Autodesk Fusion 360 part; units mm, degrees
(part 3 of 4)
sketch "Ultra96-V2" plane through (0, -0.5, 0) normal (0, -1, 0) x (1, 0, 0) in component "Card Plate"
  circle A0 centre (18.5, 38.5) radius 1.35
  circle A1 centre (18.5, -38.5) radius 1.35
  circle A2 centre (4, -38.5) radius 1.35
  circle A3 centre (4, 38.5) radius 1.35
  circle A4 centre (50, -38.5) radius 1.35
  circle A5 centre (81.5, 38.5) radius 1.35
  circle A6 centre (50, 38.5) radius 1.35
  circle A7 centre (81.5, -38.5) radius 1.35
  circle A8 centre (75, 46) radius 1.35
  circle A9 centre (17, -46) radius 1.35
  circle A10 centre (17, 46) radius 1.35
  circle A11 centre (75, -46) radius 1.35
  circle A12 centre (81.5, 24.5) radius 1.35
  circle A13 centre (81.5, -24.5) radius 1.35
  circle A14 centre (23.5, 24.5) radius 1.35
  circle A15 centre (23.5, -24.5) radius 1.35
  line L0 (100, 52) -> (15, 52)
  line L1 (15, 52) -> (15, 50)
  line L2 (15, 50) -> (0, 50)
  line L3 (0, 50) -> (0, -50)
  line L4 (0, -50) -> (15, -50)
  line L5 (15, -50) -> (15, -52)
  line L6 (15, -52) -> (100, -52)
  line L7 (100, -52) -> (100, 52)
  line L8 (0, 42.5) -> (54, 42.5) construction
  line L9 (54, 42.5) -> (54, -42.5) construction
  line L10 (54, -42.5) -> (0, -42.5) construction
  line L11 (0, -42.5) -> (0, 42.5) construction
  circle A16 centre (6, 17.5) radius 1.35
  circle A17 centre (48, 17.5) radius 1.35
  circle A18 centre (48, -24.5) radius 1.35
  circle A19 centre (6, -24.5) radius 1.35
  line L12 (6, 17.5) -> (48, 17.5) construction
  line L13 (48, 17.5) -> (48, -24.5) construction
  line L14 (48, -24.5) -> (6, -24.5) construction
  line L15 (6, -24.5) -> (6, 17.5) construction
  line L16 (31.5836, -52) -> (31.5836, -42.5) construction
  line L17 (34.961, 42.5) -> (34.961, 52) construction
  dimension "d222" = 54
  dimension "d223" = 85
  dimension "d224" = 2.7
  dimension "d225" = 2.7
  dimension "d226" = 2.7
  dimension "d227" = 2.7
  dimension "d228" = 42
  dimension "d229" = 42
  dimension "d231" = 18
  dimension "d232" = 6
  constraint horizontal L8
  constraint vertical L9
  constraint horizontal L10
  constraint vertical L11
  constraint collinear L3 L11
  constraint coincident A16.centre L12.start
  constraint coincident A17.centre L12.end
  constraint coincident A18.centre L13.end
  constraint vertical L13
  constraint coincident A19.centre L14.end
  constraint vertical L15
  constraint horizontal L12
  constraint horizontal L14
  constraint coincident L6 L16.start
  constraint coincident L10 L16.end
  constraint perpendicular L10 L16
  constraint coincident L8 L17.start
  constraint coincident L0 L17.end
  constraint perpendicular L0 L17
  constraint equal L16 L17
  measures "d222" distance of L8.start L8.end
  measures "d223" distance of L8.start L10.end
  measures "d224" diameter of A16
  measures "d225" diameter of A17
  measures "d226" diameter of A19
  measures "d227" diameter of A18
  measures "d228" distance of A16.centre A17.centre
  measures "d229" distance of A19.centre A16.centre
  measures "d231" distance of L10 A18.centre
  measures "d232" distance of L9 A18.centre
extrude "Extrude12" cut sketch "Ultra96-V2" against normal blind 8 contours A16 | A17 | A18 | A19 bodies 1 in component "Card Plate"
sketch "Jetson Nano" plane through (0, -0.5, 0) normal (0, -1, 0) x (1, 0, 0) in component "Card Plate"
  circle A0 centre (48, 17.5) radius 1.35
  circle A1 centre (48, -24.5) radius 1.35
  circle A2 centre (6, 17.5) radius 1.35
  circle A3 centre (6, -24.5) radius 1.35
  circle A4 centre (18.5, 38.5) radius 1.35
  circle A5 centre (18.5, -38.5) radius 1.35
  circle A6 centre (4, -38.5) radius 1.35
  circle A7 centre (4, 38.5) radius 1.35
  circle A8 centre (50, -38.5) radius 1.35
  circle A9 centre (81.5, 38.5) radius 1.35
  circle A10 centre (50, 38.5) radius 1.35
  circle A11 centre (81.5, -38.5) radius 1.35
  circle A12 centre (75, 46) radius 1.35
  circle A13 centre (17, -46) radius 1.35
  circle A14 centre (17, 46) radius 1.35
  circle A15 centre (75, -46) radius 1.35
  circle A16 centre (81.5, 24.5) radius 1.35
  circle A17 centre (81.5, -24.5) radius 1.35
  circle A18 centre (23.5, 24.5) radius 1.35
  circle A19 centre (23.5, -24.5) radius 1.35
  line L0 (100, 52) -> (15, 52)
  line L1 (15, 52) -> (15, 50)
  line L2 (15, 50) -> (0, 50)
  line L3 (0, 50) -> (0, -50)
  line L4 (0, -50) -> (15, -50)
  line L5 (15, -50) -> (15, -52)
  line L6 (15, -52) -> (100, -52)
  line L7 (100, -52) -> (100, 52)
  line L8 (0, 50) -> (79, 50) construction
  line L9 (79, 50) -> (79, -50) construction
  line L10 (79, -50) -> (0, -50) construction
  line L11 (0, -50) -> (0, 50) construction
  line L12 (29.4049, 50) -> (29.4049, 52) construction
  line L13 (32.781, -50) -> (32.781, -52) construction
  circle A20 centre (17, 46) radius 1.35
  circle A21 centre (75, 46) radius 1.35
  circle A22 centre (17, -40) radius 1.35
  circle A23 centre (75, -40) radius 1.35
  line L14 (17, 46) -> (75, 46) construction
  line L15 (75, 46) -> (75, -40) construction
  line L16 (75, -40) -> (17, -40) construction
  line L17 (17, -40) -> (17, 46) construction
  dimension "d235" = 79
  dimension "d236" = 100
  dimension "d237" = 2.7
  dimension "d238" = 2.7
  dimension "d239" = 2.7
  dimension "d240" = 2.7
  dimension "d241" = 17
  dimension "d242" = 4
  dimension "d243" = 86
  dimension "d244" = 58
  constraint horizontal L8
  constraint vertical L9
  constraint horizontal L10
  constraint vertical L11
  constraint coincident L8 L12.start
  constraint coincident L0 L12.end
  constraint perpendicular L0 L12
  constraint coincident L10 L13.start
  constraint coincident L6 L13.end
  constraint perpendicular L6 L13
  constraint equal L12 L13
  constraint collinear L3 L11
  constraint coincident A14.centre A20.centre
  constraint coincident A12.centre A21.centre
  constraint coincident A23.centre L15.end
  constraint coincident A22.centre L16.end
  constraint horizontal L14
  constraint vertical L15
  constraint vertical L17
  constraint horizontal L16
  measures "d235" distance of L2.end L8.end
  measures "d236" distance of L2.end L3.end
  measures "d237" diameter of A20
  measures "d238" diameter of A21
  measures "d239" diameter of A22
  measures "d240" diameter of A23
  measures "d241" distance of L11 A14.centre
  measures "d242" distance of L8 A14.centre
  measures "d243" distance of A14.centre A22.centre
  measures "d244" distance of A14.centre A12.centre
extrude "Extrude13" cut sketch "Jetson Nano" against normal blind 12 contours A5 A22 | A23 picked at (17.0516, -39.9573) bodies 1 in component "Card Plate"
sketch "SolidRun Hummingboard" plane through (0, -0.5, 0) normal (0, -1, 0) x (1, 0, 0) in component "Card Plate"
  line L0 (100, 52) -> (15, 52)
  line L1 (15, 52) -> (15, 50)
  line L2 (15, 50) -> (0, 50)
  line L3 (0, 50) -> (0, -50)
  line L4 (0, -50) -> (15, -50)
  line L5 (15, -50) -> (15, -52)
  line L6 (15, -52) -> (100, -52)
  line L7 (100, -52) -> (100, 52)
  circle A0 centre (23.5, -24.5) radius 1.35
  circle A1 centre (23.5, 24.5) radius 1.35
  circle A2 centre (81.5, -24.5) radius 1.35
  circle A3 centre (81.5, 24.5) radius 1.35
  circle A4 centre (75, -46) radius 1.35
  circle A5 centre (17, 46) radius 1.35
  circle A6 centre (17, -46) radius 1.35
  circle A7 centre (75, 46) radius 1.35
  circle A8 centre (81.5, -38.5) radius 1.35
  circle A9 centre (50, 38.5) radius 1.35
  circle A10 centre (81.5, 38.5) radius 1.35
  circle A11 centre (50, -38.5) radius 1.35
  circle A12 centre (4, 38.5) radius 1.35
  circle A13 centre (4, -38.5) radius 1.35
  arc A14 (17.1594, -38.6594) -> (18.3406, -39.8406) centre (17, -40) ccw
  arc A15 (18.3406, -39.8406) -> (17.1594, -38.6594) centre (18.5, -38.5) ccw
  circle A16 centre (18.5, 38.5) radius 1.35
  circle A17 centre (6, -24.5) radius 1.35
  circle A18 centre (6, 17.5) radius 1.35
  circle A19 centre (48, -24.5) radius 1.35
  circle A20 centre (48, 17.5) radius 1.35
  circle A21 centre (75, -40) radius 1.35
  line L8 (0, 50.959) -> (73, 50.959) construction
  line L9 (73, 50.959) -> (73, -49.041) construction
  line L10 (73, -49.041) -> (0, -49.041) construction
  line L11 (0, -49.041) -> (0, 50.959) construction
  circle A22 centre (2.838, 46.861) radius 1.35
  circle A23 centre (68.73, 48.639) radius 1.35
  circle A24 centre (68.73, -46.861) radius 1.35
  circle A25 centre (4.33, -46.861) radius 1.35
  line L12 (2.838, 46.861) -> (2.838, 50) construction
  line L13 (4.33, -46.861) -> (4.33, -50) construction
  dimension "d247" = 73
  dimension "d248" = 100
  dimension "d249" = 2.7
  dimension "d250" = 2.7
  dimension "d251" = 2.7
  dimension "d252" = 2.7
  dimension "d253" = 2.838
  dimension "d254" = 4.098
  dimension "d255" = 4.27
  dimension "d256" = 2.32
  dimension "d257" = 4.27
  dimension "d258" = 2.18
  dimension "d259" = 4.33
  dimension "d260" = 2.18
  constraint horizontal L8
  constraint vertical L9
  constraint horizontal L10
  constraint vertical L11
  constraint collinear L3 L11
  constraint coincident A22.centre L12.start
  constraint coincident L2 L12.end
  constraint perpendicular L2 L12
  constraint coincident A25.centre L13.start
  constraint coincident L4 L13.end
  constraint perpendicular L4 L13
  constraint equal L12 L13
  measures "d247" distance of L8.start L8.end
  measures "d248" distance of L8.start L10.end
  measures "d249" diameter of A22
  measures "d250" diameter of A23
  measures "d251" diameter of A24
  measures "d252" diameter of A25
  measures "d253" distance of L11 A22.centre
  measures "d254" distance of L8 A22.centre
  measures "d255" distance of L9 A23.centre
  measures "d256" distance of L8 A23.centre
  measures "d257" distance of L9 A24.centre
  measures "d258" distance of L10 A24.centre
  measures "d259" distance of L11 A25.centre
  measures "d260" distance of L10 A25.centre
extrude "Extrude14" cut sketch "SolidRun Hummingboard" against normal blind 55 contours A22 | A23 | A24 | A25 bodies 1 in component "Card Plate"
sketch "Cutout - Broad" plane through (0, -0.5, 0) normal (0, -1, 0) x (1, 0, 0) in component "Card Plate"
  circle A0 centre (68.73, 48.639) radius 1.35
  circle A1 centre (4.33, -46.861) radius 1.35
  circle A2 centre (2.838, 46.861) radius 1.35
  circle A3 centre (68.73, -46.861) radius 1.35
  line L0 (100, 52) -> (15, 52)
  line L1 (15, 52) -> (15, 50)
  line L2 (15, 50) -> (0, 50)
  line L3 (0, 50) -> (0, -50)
  line L4 (0, -50) -> (15, -50)
  line L5 (15, -50) -> (15, -52)
  line L6 (15, -52) -> (100, -52)
  line L7 (100, -52) -> (100, 52)
  circle A4 centre (23.5, -24.5) radius 1.35
  circle A5 centre (23.5, 24.5) radius 1.35
  circle A6 centre (81.5, -24.5) radius 1.35
  circle A7 centre (81.5, 24.5) radius 1.35
  circle A8 centre (75, -46) radius 1.35
  circle A9 centre (17, 46) radius 1.35
  circle A10 centre (17, -46) radius 1.35
  circle A11 centre (75, 46) radius 1.35
  circle A12 centre (81.5, -38.5) radius 1.35
  circle A13 centre (50, 38.5) radius 1.35
  circle A14 centre (81.5, 38.5) radius 1.35
  circle A15 centre (50, -38.5) radius 1.35
  circle A16 centre (4, 38.5) radius 1.35
  circle A17 centre (4, -38.5) radius 1.35
  arc A18 (17.1594, -38.6594) -> (18.3406, -39.8406) centre (17, -40) ccw
  arc A19 (18.3406, -39.8406) -> (17.1594, -38.6594) centre (18.5, -38.5) ccw
  circle A20 centre (18.5, 38.5) radius 1.35
  circle A21 centre (6, -24.5) radius 1.35
  circle A22 centre (6, 17.5) radius 1.35
  circle A23 centre (48, -24.5) radius 1.35
  circle A24 centre (48, 17.5) radius 1.35
  circle A25 centre (75, -40) radius 1.35
  line L8 (11, -33.5) -> (18.5, -33.5)
  line L9 (18.5, -33.5) -> (18.5, -19.5)
  line L10 (18.5, -19.5) -> (28.5, -19.5)
  line L11 (28.5, -19.5) -> (28.5, -47)
  line L12 (28.5, -47) -> (43, -47)
  line L13 (43, -47) -> (43, -19.5)
  line L14 (43, -19.5) -> (55, -19.5)
  line L15 (55, -19.5) -> (55, -47)
  line L16 (55, -47) -> (63.73, -47)
  line L17 (63.73, -47) -> (63.73, -44.9205)
  line L18 (63.73, -44.9205) -> (76.5, -30.9468)
  line L19 (76.5, -30.9468) -> (76.5, -18.1196)
  line L20 (76.5, -18.1196) -> (86.5, -18.1196)
  line L21 (86.5, -18.1196) -> (86.5, -47)
  line L22 (86.5, -47) -> (95, -47)
  line L23 (95, -47) -> (95, 47)
  line L24 (95, 47) -> (86.5, 47)
  line L25 (86.5, 47) -> (86.5, 19.5)
  line L26 (86.5, 19.5) -> (76.5, 19.5)
  line L27 (76.5, 19.5) -> (76.5, 39.9438)
  line L28 (76.5, 39.9438) -> (59.7352, 47)
  line L29 (59.7352, 47) -> (55, 47)
  line L30 (55, 47) -> (55, 12.5)
  line L31 (55, 12.5) -> (43, 12.5)
  line L32 (43, 12.5) -> (43, 47)
  line L33 (43, 47) -> (28.5, 47)
  line L34 (28.5, 47) -> (28.5, 19.5)
  line L35 (28.5, 19.5) -> (18.5, 19.5)
  line L36 (18.5, 19.5) -> (18.5, 33.5)
  line L37 (18.5, 33.5) -> (11, 33.5)
  line L38 (100, 52) -> (100, -52)
  line L39 (15, 52) -> (100, 52)
  line L40 (100, -52) -> (15, -52)
  line L41 (11, -33.5) -> (11, -19.5)
  line L42 (11, -19.5) -> (5, -19.5)
  line L43 (5, -19.5) -> (5, 12.5)
  line L44 (5, 12.5) -> (11, 12.5)
  line L45 (11, 12.5) -> (11, 33.5)
  dimension "d287" = 5
  dimension "d288" = 5
  dimension "d289" = 5
  dimension "d290" = 5
  dimension "d291" = 5
  dimension "d292" = 5
  dimension "d293" = 5
  dimension "d294" = 5
  dimension "d295" = 5
  dimension "d296" = 5
  dimension "d297" = 5
  dimension "d298" = 5
  dimension "d299" = 5
  dimension "d300" = 5
  dimension "d301" = 5
  dimension "d302" = 5
  dimension "d303" = 5
  dimension "d306" = 5
  dimension "d307" = 5
  dimension "d308" = 5
  dimension "d309" = 5
  dimension "d310" = 5
  dimension "d311" = 5
  dimension "d312" = 5
  dimension "d313" = 5
  dimension "d314" = 5
  dimension "d315" = 5
  dimension "d316" = 5
  dimension "d317" = 5
  dimension "d318" = 5
  dimension "d319" = 5
  dimension "d320" = 5
  dimension "d321" = 5
  dimension "d322" = 5
  dimension "d323" = 5
  dimension "d324" = 5
  constraint perpendicular L8 L9
  constraint perpendicular L9 L10
  constraint perpendicular L10 L11
  constraint perpendicular L11 L12
  constraint perpendicular L12 L13
  constraint perpendicular L13 L14
  constraint perpendicular L12 L15
  constraint perpendicular L15 L16
  constraint perpendicular L16 L17
  constraint perpendicular L16 L19
  constraint perpendicular L19 L20
  constraint perpendicular L20 L21
  constraint perpendicular L21 L22
  constraint perpendicular L22 L23
  constraint perpendicular L23 L24
  constraint perpendicular L24 L25
  constraint perpendicular L25 L26
  constraint perpendicular L26 L27
  constraint perpendicular L27 L29
  constraint perpendicular L29 L30
  constraint perpendicular L30 L31
  constraint perpendicular L29 L32
  constraint perpendicular L32 L33
  constraint perpendicular L33 L34
  constraint perpendicular L34 L35
  constraint perpendicular L33 L36
  constraint perpendicular L36 L37
  constraint perpendicular L8 L41
  constraint perpendicular L41 L42
  constraint perpendicular L42 L43
  constraint perpendicular L43 L44
  constraint perpendicular L37 L45
  measures "d287" distance of L23 L38
  measures "d288" distance of A6.centre L21
  measures "d289" distance of A7.centre L25
  measures "d290" distance of A7.centre L27
  measures "d291" distance of L29 L39
  measures "d292" distance of L33 L39
  measures "d293" distance of L16 L40
  measures "d294" distance of L12 L40
  measures "d295" distance of A3.centre L17
  measures "d296" distance of A6.centre L19
  measures "d297" distance of A25.centre L18
  measures "d298" distance of A3.centre L18
  measures "d299" distance of A13.centre L30
  measures "d300" distance of A24.centre L32
  measures "d301" distance of A5.centre L34
  measures "d302" distance of A5.centre L35
  measures "d303" distance of A20.centre L37
  measures "d306" distance of A4.centre L11
  measures "d307" distance of A15.centre L15
  measures "d308" distance of A23.centre L13
  measures "d309" distance of A4.centre L9
  measures "d310" distance of A4.centre L10
  measures "d311" distance of A19.centre L8
  measures "d312" distance of A0.centre L28
  measures "d313" distance of A11.centre L28
  measures "d314" distance of A7.centre L26
  measures "d315" distance of A24.centre L31
  measures "d316" distance of A23.centre L14
  measures "d317" distance of L22 L40
  measures "d318" distance of L24 L39
  measures "d319" distance of A22.centre L45
  measures "d320" distance of L3 L43
  measures "d321" distance of A21.centre L42
  measures "d322" distance of A21.centre L41
  measures "d323" distance of A5.centre L36
  measures "d324" distance of A22.centre L44
extrude "Extrude15" cut sketch "Cutout - Broad" against normal blind 20 contours L8 L9 L10 L11 L12 L13 L14 L15 L16 L17 L18 L19 L20 L21 L22 L23 L24 L25 L26 L27 L28 L29 L30 L31 L32 L33 L34 L35 L36 L37 L41 L42 L43 L44 L45 bodies 1 in component "Card Plate"
sketch "Cutout - Supports" plane through (0, -0.5, 0) normal (0, -1, 0) x (1, 0, 0) in component "Card Plate"
  line L0 (18.5, -19.5) -> (18.5, -33.5)
  line L1 (18.5, -33.5) -> (11, -33.5)
  line L2 (11, -33.5) -> (11, -19.5)
  line L3 (11, -19.5) -> (5, -19.5)
  line L4 (5, -19.5) -> (5, 12.5)
  line L5 (5, 12.5) -> (11, 12.5)
  line L6 (11, 12.5) -> (11, 33.5)
  line L7 (11, 33.5) -> (18.5, 33.5)
  line L8 (18.5, 33.5) -> (18.5, 19.5)
  line L9 (18.5, 19.5) -> (28.5, 19.5)
  line L10 (28.5, 19.5) -> (28.5, 47)
  line L11 (28.5, 47) -> (43, 47)
  line L12 (43, 47) -> (43, 12.5)
  line L13 (43, 12.5) -> (55, 12.5)
  line L14 (55, 12.5) -> (55, 47)
  line L15 (55, 47) -> (59.7352, 47)
  line L16 (59.7352, 47) -> (76.5, 39.9438)
  line L17 (76.5, 39.9438) -> (76.5, 19.5)
  line L18 (76.5, 19.5) -> (86.5, 19.5)
  line L19 (86.5, 19.5) -> (86.5, 47)
  line L20 (86.5, 47) -> (95, 47)
  line L21 (95, 47) -> (95, -47)
  line L22 (95, -47) -> (86.5, -47)
  line L23 (86.5, -47) -> (86.5, -18.1196)
  line L24 (86.5, -18.1196) -> (76.5, -18.1196)
  line L25 (76.5, -18.1196) -> (76.5, -30.9468)
  line L26 (76.5, -30.9468) -> (63.73, -44.9205)
  line L27 (63.73, -44.9205) -> (63.73, -47)
  line L28 (63.73, -47) -> (55, -47)
  line L29 (55, -47) -> (55, -19.5)
  line L30 (55, -19.5) -> (43, -19.5)
  line L31 (43, -19.5) -> (43, -47)
  line L32 (43, -47) -> (28.5, -47)
  line L33 (28.5, -47) -> (28.5, -19.5)
  line L34 (28.5, -19.5) -> (18.5, -19.5)
  circle A0 centre (68.73, 48.639) radius 1.35
  circle A1 centre (4.33, -46.861) radius 1.35
  circle A2 centre (2.838, 46.861) radius 1.35
  circle A3 centre (68.73, -46.861) radius 1.35
  line L35 (100, 52) -> (15, 52)
  line L36 (15, 52) -> (15, 50)
  line L37 (15, 50) -> (0, 50)
  line L38 (0, 50) -> (0, -50)
  line L39 (0, -50) -> (15, -50)
  line L40 (15, -50) -> (15, -52)
  line L41 (15, -52) -> (100, -52)
  line L42 (100, -52) -> (100, 52)
  circle A4 centre (23.5, -24.5) radius 1.35
  circle A5 centre (23.5, 24.5) radius 1.35
  circle A6 centre (81.5, -24.5) radius 1.35
  circle A7 centre (81.5, 24.5) radius 1.35
  circle A8 centre (75, -46) radius 1.35
  circle A9 centre (17, 46) radius 1.35
  circle A10 centre (17, -46) radius 1.35
  circle A11 centre (75, 46) radius 1.35
  circle A12 centre (81.5, -38.5) radius 1.35
  circle A13 centre (50, 38.5) radius 1.35
  circle A14 centre (81.5, 38.5) radius 1.35
  circle A15 centre (50, -38.5) radius 1.35
  circle A16 centre (4, 38.5) radius 1.35
  circle A17 centre (4, -38.5) radius 1.35
  arc A18 (17.1594, -38.6594) -> (18.3406, -39.8406) centre (17, -40) ccw
  arc A19 (18.3406, -39.8406) -> (17.1594, -38.6594) centre (18.5, -38.5) ccw
  circle A20 centre (18.5, 38.5) radius 1.35
  circle A21 centre (6, -24.5) radius 1.35
  circle A22 centre (6, 17.5) radius 1.35
  circle A23 centre (48, -24.5) radius 1.35
  circle A24 centre (48, 17.5) radius 1.35
  circle A25 centre (75, -40) radius 1.35
  line L43 (18.5, 19.5) -> (11, 19.5)
  line L44 (28.5, 19.5) -> (43, 12.5)
  line L45 (55, 12.5) -> (76.5, 19.5)
  line L46 (86.5, 19.5) -> (95, 19.5)
  line L47 (11, -19.5) -> (18.5, -19.5)
  line L48 (28.5, -19.5) -> (43, -19.5)
  line L49 (55, -19.5) -> (76.5, -18.1196)
  line L50 (86.5, -18.1196) -> (95, -18.1196)
  line L51 (43, 12.5) -> (43, -19.5)
  line L52 (55, 12.5) -> (55, -19.5)
  line L53 (76.5, 19.5) -> (76.5, -18.1196)
  line L54 (28.5, 19.5) -> (28.5, -19.5)
  line L55 (18.5, -19.5) -> (18.5, 19.5)
  line L56 (11, 12.5) -> (11, -19.5)
  line L57 (0, 0) -> (95, 0) construction
  line L58 (86.5, 19.5) -> (86.5, -18.1196)
  line L59 (53, 12.5) -> (53, -19.5)
  line L60 (45, 12.5) -> (45, -19.5)
  line L61 (54.3808, 14.4017) -> (75.8808, 21.4017)
  line L62 (75.8808, 21.4017) -> (76.746, 21.6834)
  line L63 (86.5, 21.5) -> (95, 21.5)
  line L64 (29.3695, 21.3011) -> (43.8695, 14.3011)
  line L65 (29.3695, 21.3011) -> (26.7566, 22.5625)
  line L66 (18.5, 21.5) -> (11, 21.5)
  line L67 (11, -21.5) -> (18.5, -21.5)
  line L68 (28.5, -21.5) -> (43, -21.5)
  line L69 (55.1281, -21.4959) -> (76.6281, -20.1155)
  line L70 (55.1281, -21.4959) -> (53.7975, -21.5813)
  line L71 (86.5, -20.1196) -> (95, -20.1196)
  line L72 (84.5, 19.5) -> (84.5, -18.1196)
  line L73 (78.5, 19.5) -> (78.5, -18.1196)
  line L74 (0, -1) -> (95, -1)
  line L75 (0, 1) -> (95, 1)
  line L76 (9, 12.5) -> (9, -19.5)
  line L77 (20.5, -19.5) -> (20.5, 19.5)
  line L78 (26.5, 19.5) -> (26.5, -19.5)
  dimension "d327" = 2
  dimension "d328" = -2
  dimension "d329" = -2
  dimension "d330" = -2
  dimension "d331" = -2
  dimension "d332" = 2
  dimension "d333" = 2
  dimension "d334" = 2
  dimension "d335" = 2
  dimension "d336" = 2
  dimension "d337" = 2
  dimension "d338" = -2
  dimension "d339" = 1
  dimension "d340" = -1
  dimension "d341" = 2
  dimension "d342" = 2
  dimension "d343" = 2
  constraint coincident L8.end L9.start
  constraint coincident L6 L43.end
  constraint perpendicular L6 L43
  constraint coincident L9.end L10.start
  constraint coincident L12.end L13.start
  constraint coincident L13.end L14.start
  constraint coincident L17.end L18.start
  constraint coincident L18.end L19.start
  constraint coincident L21 L46.end
  constraint perpendicular L21 L46
  constraint coincident L2.end L3.start
  constraint coincident L0.start L34.end
  constraint coincident L33.end L34.start
  constraint coincident L30.end L31.start
  constraint coincident L29.end L30.start
  constraint coincident L24.end L25.start
  constraint coincident L23.end L24.start
  constraint coincident L21 L50.end
  constraint perpendicular L21 L50
  constraint coincident L5.end L6.start
  constraint coincident L57.start origin
  constraint midpoint L21 L57.end
  constraint parallel L61 L62
  constraint parallel L64 L65
  constraint parallel L69 L70
extrude "Extrude16" add sketch "Cutout - Supports" against normal blind 2.5 contours L34 L55 L74 L77 | L0 L2 L47 L67 | L3 L56 L74 L76 | L55 L56 L74 L75 | L55 L74 L75 L77 | L34 L54 L74 L78 | L74 L75 L77 L78 | L56 L74 L75 L76 | L9 L55 L75 L77 | L31 L33 L48 L68 | L54 L74 L75 L78 | L4 L74 L75 L76 | L5 L56 L75 L76 | L6 L8 L43 L66 | L30 L51 L60 L74 | L51 L54 L74 L75 | L9 L54 L75 L78 | L51 L60 L74 L75 | L30 L52 L59 L74 | L59 L60 L74 L75 | L13 L51 L60 L75 | L10 L12 L44 L64 L65 | L25 L29 L49 L69 L70 | L52 L59 L74 L75 | L24 L53 L73 L74 | L52 L53 L74 L75 | L13 L52 L59 L75 | L53 L73 L74 L75 | L24 L58 L72 L74 | L72 L73 L74 L75 | L18 L53 L73 L75 | L14 L17 L45 L61 L62 | L21 L23 L50 L71 | L58 L72 L74 L75 | L21 L58 L74 L75 | L18 L58 L72 L75 | L19 L21 L46 L63 bodies 1 in component "Card Plate"
sketch "Cutout - 2nd Round" plane through (0, -0.5, 0) normal (0, -1, 0) x (1, 0, 0) in component "Card Plate"
  line L0 (76.5, -20.1237) -> (76.5, -30.9468)
  line L1 (76.5, -30.9468) -> (63.73, -44.9205)
  line L2 (63.73, -44.9205) -> (63.73, -47)
  line L3 (63.73, -47) -> (55, -47)
  line L4 (55, -47) -> (55, -21.5041)
  line L5 (55, -21.5041) -> (76.5, -20.1237)
  line L6 (76.5, -18.1196) -> (55, -19.5)
  line L7 (55, -19.5) -> (55, -1)
  line L8 (55, -1) -> (76.5, -1)
  line L9 (76.5, -1) -> (76.5, -18.1196)
  line L10 (18.5, -21.5) -> (18.5, -33.5)
  line L11 (18.5, -33.5) -> (11, -33.5)
  line L12 (11, -33.5) -> (11, -21.5)
  line L13 (11, -21.5) -> (18.5, -21.5)
  line L14 (18.5, -19.5) -> (11, -19.5)
  line L15 (11, -19.5) -> (11, -1)
  line L16 (11, -1) -> (18.5, -1)
  line L17 (18.5, -1) -> (18.5, -19.5)
  line L18 (11, 21.5) -> (11, 33.5)
  line L19 (11, 33.5) -> (18.5, 33.5)
  line L20 (18.5, 33.5) -> (18.5, 21.5)
  line L21 (18.5, 21.5) -> (11, 21.5)
  line L22 (55, 14.6033) -> (55, 47)
  line L23 (55, 47) -> (59.7352, 47)
  line L24 (59.7352, 47) -> (76.5, 39.9438)
  line L25 (76.5, 39.9438) -> (76.5, 21.6033)
  line L26 (76.5, 21.6033) -> (55, 14.6033)
  line L27 (55, 12.5) -> (76.5, 19.5)
  line L28 (76.5, 19.5) -> (76.5, 1)
  line L29 (76.5, 1) -> (55, 1)
  line L30 (55, 1) -> (55, 12.5)
  line L31 (43, -21.5) -> (43, -47)
  line L32 (43, -47) -> (28.5, -47)
  line L33 (28.5, -47) -> (28.5, -21.5)
  line L34 (28.5, -21.5) -> (43, -21.5)
  line L35 (43, -19.5) -> (28.5, -19.5)
  line L36 (28.5, -19.5) -> (28.5, -1)
  line L37 (28.5, -1) -> (43, -1)
  line L38 (43, -1) -> (43, -19.5)
  line L39 (95, -20.1196) -> (95, -47)
  line L40 (95, -47) -> (86.5, -47)
  line L41 (86.5, -47) -> (86.5, -20.1196)
  line L42 (86.5, -20.1196) -> (95, -20.1196)
  line L43 (28.5, 21.7209) -> (28.5, 47)
  line L44 (28.5, 47) -> (43, 47)
  line L45 (43, 47) -> (43, 14.7209)
  line L46 (43, 14.7209) -> (28.5, 21.7209)
  line L47 (28.5, 19.5) -> (43, 12.5)
  line L48 (43, 12.5) -> (43, 1)
  line L49 (43, 1) -> (28.5, 1)
  line L50 (28.5, 1) -> (28.5, 19.5)
  line L51 (26.5, 19.5) -> (26.5, 1)
  line L52 (26.5, 1) -> (20.5, 1)
  line L53 (20.5, 1) -> (20.5, 19.5)
  line L54 (20.5, 19.5) -> (26.5, 19.5)
  line L55 (11, 19.5) -> (18.5, 19.5)
  line L56 (18.5, 19.5) -> (18.5, 1)
  line L57 (18.5, 1) -> (11, 1)
  line L58 (11, 1) -> (11, 19.5)
  line L59 (9, 12.5) -> (9, 1)
  line L60 (9, 1) -> (5, 1)
  line L61 (5, 1) -> (5, 12.5)
  line L62 (5, 12.5) -> (9, 12.5)
  line L63 (5, -1) -> (9, -1)
  line L64 (9, -1) -> (9, -19.5)
  line L65 (9, -19.5) -> (5, -19.5)
  line L66 (5, -19.5) -> (5, -1)
  line L67 (20.5, -19.5) -> (20.5, -1)
  line L68 (20.5, -1) -> (26.5, -1)
  line L69 (26.5, -1) -> (26.5, -19.5)
  line L70 (26.5, -19.5) -> (20.5, -19.5)
  line L71 (45, -19.5) -> (45, -1)
  line L72 (45, -1) -> (53, -1)
  line L73 (53, -1) -> (53, -19.5)
  line L74 (53, -19.5) -> (45, -19.5)
  line L75 (78.5, -18.1196) -> (78.5, -1)
  line L76 (78.5, -1) -> (84.5, -1)
  line L77 (84.5, -1) -> (84.5, -18.1196)
  line L78 (84.5, -18.1196) -> (78.5, -18.1196)
  line L79 (95, -18.1196) -> (86.5, -18.1196)
  line L80 (86.5, -18.1196) -> (86.5, -1)
  line L81 (86.5, -1) -> (95, -1)
  line L82 (95, -1) -> (95, -18.1196)
  line L83 (78.5, 19.5) -> (84.5, 19.5)
  line L84 (84.5, 19.5) -> (84.5, 1)
  line L85 (84.5, 1) -> (78.5, 1)
  line L86 (78.5, 1) -> (78.5, 19.5)
  line L87 (53, 12.5) -> (53, 1)
  line L88 (53, 1) -> (45, 1)
  line L89 (45, 1) -> (45, 12.5)
  line L90 (45, 12.5) -> (53, 12.5)
  line L91 (95, 1) -> (86.5, 1)
  line L92 (86.5, 1) -> (86.5, 19.5)
  line L93 (86.5, 19.5) -> (95, 19.5)
  line L94 (95, 19.5) -> (95, 1)
  line L95 (95, 21.5) -> (86.5, 21.5)
  line L96 (86.5, 21.5) -> (86.5, 47)
  line L97 (86.5, 47) -> (95, 47)
  line L98 (95, 47) -> (95, 21.5)
  circle A0 centre (68.73, 48.639) radius 1.35
  circle A1 centre (4.33, -46.861) radius 1.35
  circle A2 centre (2.838, 46.861) radius 1.35
  circle A3 centre (68.73, -46.861) radius 1.35
  line L99 (100, 52) -> (15, 52)
  line L100 (15, 52) -> (15, 50)
  line L101 (15, 50) -> (0, 50)
  line L102 (0, 50) -> (0, -50)
  line L103 (0, -50) -> (15, -50)
  line L104 (15, -50) -> (15, -52)
  line L105 (15, -52) -> (100, -52)
  line L106 (100, -52) -> (100, 52)
  circle A4 centre (23.5, -24.5) radius 1.35
  circle A5 centre (23.5, 24.5) radius 1.35
  circle A6 centre (81.5, -24.5) radius 1.35
  circle A7 centre (81.5, 24.5) radius 1.35
  circle A8 centre (75, -46) radius 1.35
  circle A9 centre (17, 46) radius 1.35
  circle A10 centre (17, -46) radius 1.35
  circle A11 centre (75, 46) radius 1.35
  circle A12 centre (81.5, -38.5) radius 1.35
  circle A13 centre (50, 38.5) radius 1.35
  circle A14 centre (81.5, 38.5) radius 1.35
  circle A15 centre (50, -38.5) radius 1.35
  circle A16 centre (4, 38.5) radius 1.35
  circle A17 centre (4, -38.5) radius 1.35
  arc A18 (17.1594, -38.6594) -> (18.3406, -39.8406) centre (17, -40) ccw
  arc A19 (18.3406, -39.8406) -> (17.1594, -38.6594) centre (18.5, -38.5) ccw
  circle A20 centre (18.5, 38.5) radius 1.35
  circle A21 centre (6, -24.5) radius 1.35
  circle A22 centre (6, 17.5) radius 1.35
  circle A23 centre (48, -24.5) radius 1.35
  circle A24 centre (48, 17.5) radius 1.35
  circle A25 centre (75, -40) radius 1.35
  line L107 (5, 33.5) -> (9, 33.5)
  line L108 (9, 33.5) -> (9, 22.5)
  line L109 (9, 22.5) -> (5, 22.5)
  line L110 (5, 22.5) -> (5, 33.5)
  line L111 (20.5, 33.5) -> (26.5, 33.5)
  line L112 (26.5, 33.5) -> (26.5, 29.5)
  line L113 (26.5, 29.5) -> (20.5, 29.5)
  line L114 (20.5, 29.5) -> (20.5, 33.5)
  line L115 (45, 33.5) -> (53, 33.5)
  line L116 (53, 33.5) -> (53, 22.5)
  line L117 (53, 22.5) -> (45, 22.5)
  line L118 (45, 22.5) -> (45, 33.5)
  line L119 (78.5, 33.5) -> (84.5, 33.5)
  line L120 (84.5, 33.5) -> (84.5, 29.5)
  line L121 (84.5, 29.5) -> (78.5, 29.5)
  line L122 (78.5, 29.5) -> (78.5, 33.5)
  line L123 (80, 47) -> (84.5, 47)
  line L124 (84.5, 47) -> (84.5, 43.5)
  line L125 (84.5, 43.5) -> (80, 43.5)
  line L126 (80, 43.5) -> (80, 47)
  line L127 (45, 47) -> (53, 47)
  line L128 (53, 47) -> (53, 43.5)
  line L129 (53, 43.5) -> (45, 43.5)
  line L130 (45, 43.5) -> (45, 47)
  line L131 (45, -29.5) -> (53, -29.5)
  line L132 (53, -29.5) -> (53, -33.5)
  line L133 (53, -33.5) -> (45, -33.5)
  line L134 (45, -33.5) -> (45, -29.5)
  line L135 (78.5, -29.5) -> (84.5, -29.5)
  line L136 (84.5, -29.5) -> (84.5, -33.5)
  line L137 (84.5, -33.5) -> (78.5, -33.5)
  line L138 (78.5, -33.5) -> (78.5, -29.5)
  line L139 (80, -43.5) -> (84.5, -43.5)
  line L140 (84.5, -43.5) -> (84.5, -47)
  line L141 (84.5, -47) -> (80, -47)
  line L142 (80, -47) -> (80, -43.5)
  line L143 (45, -43.5) -> (53, -43.5)
  line L144 (53, -43.5) -> (53, -47)
  line L145 (53, -47) -> (45, -47)
  line L146 (45, -47) -> (45, -43.5)
  line L147 (26.5, -29.5) -> (23.5, -29.5)
  line L148 (23.5, -29.5) -> (23.5, -47)
  line L149 (23.5, -47) -> (26.5, -47)
  line L150 (26.5, -47) -> (26.5, -29.5)
  line L151 (9, -35.5) -> (12, -35.5)
  line L152 (12, -35.5) -> (12, -45)
  line L153 (12, -45) -> (9, -45)
  line L154 (9, -45) -> (9, -35.5)
  line L155 (5, -29.5) -> (9, -29.5)
  line L156 (9, -29.5) -> (9, -33.5)
  line L157 (9, -33.5) -> (5, -33.5)
  line L158 (5, -33.5) -> (5, -29.5)
  line L159 (15, 52) -> (100, 52)
  line L160 (100, -52) -> (15, -52)
  dimension "d346" = 5
  dimension "d347" = 5
  dimension "d348" = 2
  dimension "d349" = 2
  dimension "d350" = 2
  dimension "d351" = 5
  dimension "d352" = 5
  dimension "d353" = 5
  dimension "d354" = 2
  dimension "d355" = 2
  dimension "d356" = 5
  dimension "d357" = 5
  dimension "d359" = 5
  dimension "d360" = 5
  dimension "d361" = 2
  dimension "d362" = 2
  dimension "d363" = 5
  dimension "d364" = 5
  dimension "d365" = 2
  dimension "d366" = 5
  dimension "d367" = 5
  dimension "d368" = 5
  dimension "d369" = 2
  dimension "d370" = 2
  dimension "d371" = 2
  dimension "d372" = 5
  dimension "d373" = 5
  dimension "d374" = 5
  dimension "d375" = 2
  dimension "d376" = 2
  dimension "d377" = 5
  dimension "d378" = 5
  dimension "d379" = 5
  dimension "d380" = 5
  dimension "d381" = 2
  dimension "d382" = 2
  dimension "d383" = 2
  dimension "d384" = 5
  dimension "d385" = 5
  dimension "d386" = 5
  dimension "d387" = 2
  dimension "d388" = 5
  dimension "d389" = 5
  dimension "d390" = 5
  dimension "d391" = 2
  dimension "d392" = 5
  dimension "d393" = 5
  dimension "d394" = 5
  dimension "d395" = 5
  dimension "d396" = 5
  dimension "d397" = 2
  dimension "d398" = 2
  constraint horizontal L107
  constraint vertical L108
  constraint horizontal L109
  constraint vertical L110
  constraint horizontal L111
  constraint vertical L112
  constraint horizontal L113
  constraint vertical L114
  constraint horizontal L115
  constraint vertical L116
  constraint horizontal L117
  constraint vertical L118
  constraint horizontal L119
  constraint vertical L120
  constraint horizontal L121
  constraint vertical L122
  constraint horizontal L123
  constraint vertical L124
  constraint horizontal L125
  constraint vertical L126
  constraint horizontal L127
  constraint vertical L128
  constraint horizontal L129
  constraint vertical L130
  constraint horizontal L131
  constraint vertical L132
  constraint horizontal L133
  constraint vertical L134
  constraint horizontal L135
  constraint vertical L136
  constraint horizontal L137
  constraint vertical L138
  constraint horizontal L139
  constraint vertical L140
  constraint horizontal L141
  constraint vertical L142
  constraint horizontal L143
  constraint vertical L144
  constraint horizontal L145
  constraint vertical L146
  constraint horizontal L147
  constraint vertical L148
  constraint horizontal L149
  constraint vertical L150
  constraint horizontal L151
  constraint vertical L152
  constraint horizontal L153
  constraint vertical L154
  constraint horizontal L155
  constraint vertical L156
  constraint horizontal L157
  constraint vertical L158
  measures "d346" distance of A20.centre L111
  measures "d347" distance of A5.centre L113
  measures "d348" distance of L43 L112
  measures "d349" distance of L20 L114
  measures "d350" distance of L18 L108
  measures "d351" distance of L102 L110
  measures "d352" distance of A22.centre L109
  measures "d353" distance of A16.centre L107
  measures "d354" distance of L45 L118
  measures "d355" distance of L22 L116
  measures "d356" distance of A24.centre L117
  measures "d357" distance of A13.centre L115
  measures "d359" distance of A13.centre L129
  measures "d360" distance of L127 L159
  measures "d361" distance of L45 L130
  measures "d362" distance of L22 L128
  measures "d363" distance of L123 L159
  measures "d364" distance of A14.centre L125
  measures "d365" distance of L96 L124
  measures "d366" distance of A11.centre L126
  measures "d367" distance of A6.centre L135
  measures "d368" distance of A12.centre L137
  measures "d369" distance of L41 L136
  measures "d370" distance of L0 L138
  measures "d371" distance of L41 L140
  measures "d372" distance of A8.centre L142
  measures "d373" distance of A12.centre L139
  measures "d374" distance of L141 L160
  measures "d375" distance of L4 L144
  measures "d376" distance of L31 L146
  measures "d377" distance of L105 L145
  measures "d378" distance of A15.centre L143
  measures "d379" distance of A15.centre L133
  measures "d380" distance of A23.centre L131
  measures "d381" distance of L4 L132
  measures "d382" distance of L31 L134
  measures "d383" distance of L33 L150
  measures "d384" distance of A19.centre L148
  measures "d385" distance of A4.centre L147
  measures "d386" distance of L149 L160
  measures "d387" distance of L11 L151
  measures "d388" distance of A17.centre L157
  measures "d389" distance of A21.centre L155
  measures "d390" distance of L102 L158
  measures "d391" distance of L12 L156
  measures "d392" distance of A18.centre L152
  measures "d393" distance of A17.centre L154
  measures "d394" distance of L103 L153
  measures "d395" distance of A14.centre L119
  measures "d396" distance of A7.centre L121
  measures "d397" distance of L96 L120
  measures "d398" distance of L25 L122
extrude "Extrude17" cut sketch "Cutout - 2nd Round" against normal blind 9 contours L107 L108 L109 L110 | L111 L112 L113 L114 | L115 L116 L117 L118 | L119 L120 L121 L122 | L123 L124 L125 L126 | L127 L128 L129 L130 | L131 L132 L133 L134 | L135 L136 L137 L138 | L139 L140 L141 L142 | L143 L144 L145 L146 | L147 L148 L149 L150 | L151 L152 L153 L154 | L155 L156 L157 L158 bodies 1 in component "Card Plate"
sketch "Grip Fix" plane through (0, -3, 0) normal (0, -1, 0) x (1, 0, 0) in component "Card Plate"
  line L0 (-8.25, -56.5) -> (-8.25, -55.5)
  line L1 (-8.25, -55.5) -> (-7.25, -55.5)
  line L2 (-7.25, -55.5) -> (-7.25, -56.5)
  line L3 (-7.25, -56.5) -> (-6.375, -56.5)
  line L4 (-6.375, -56.5) -> (-6.375, -55.5)
  line L5 (-6.375, -55.5) -> (-5.375, -55.5)
  line L6 (-5.375, -55.5) -> (-5.375, -56.5)
  line L7 (-5.375, -56.5) -> (-4.5, -56.5)
  line L8 (-4.5, -56.5) -> (-4.5, -55.5)
  line L9 (-4.5, -55.5) -> (-3.5, -55.5)
  line L10 (-3.5, -55.5) -> (-3.5, -56.5)
  line L11 (-3.5, -56.5) -> (-3, -56.5)
  line L12 (-3, -56.5) -> (0, -55)
  line L13 (0, -55) -> (5, -55)
  line L14 (5, -55) -> (5, -57)
  line L15 (5, -57) -> (9.5, -55)
  line L16 (9.5, -55) -> (100, -55)
  line L17 (100, -55) -> (103, -52)
  line L18 (103, -52) -> (103, 52)
  line L19 (103, 52) -> (100, 55)
  line L20 (100, 55) -> (9.5, 55)
  line L21 (9.5, 55) -> (5, 57)
  line L22 (5, 57) -> (5, 55)
  line L23 (5, 55) -> (0, 55)
  line L24 (0, 55) -> (-3, 56.5)
  line L25 (-3, 56.5) -> (-3.5, 56.5)
  line L26 (-3.5, 56.5) -> (-3.5, 55.5)
  line L27 (-3.5, 55.5) -> (-4.5, 55.5)
  line L28 (-4.5, 55.5) -> (-4.5, 56.5)
  line L29 (-4.5, 56.5) -> (-5.375, 56.5)
  line L30 (-5.375, 56.5) -> (-5.375, 55.5)
  line L31 (-5.375, 55.5) -> (-6.375, 55.5)
  line L32 (-6.375, 55.5) -> (-6.375, 56.5)
  line L33 (-6.375, 56.5) -> (-7.25, 56.5)
  line L34 (-7.25, 56.5) -> (-7.25, 55.5)
  line L35 (-7.25, 55.5) -> (-8.25, 55.5)
  line L36 (-8.25, 55.5) -> (-8.25, 56.5)
  line L37 (-8.25, 56.5) -> (-9.125, 56.5)
  line L38 (-9.125, 56.5) -> (-9.125, 55.5)
  line L39 (-9.125, 55.5) -> (-10.125, 55.5)
  line L40 (-10.125, 55.5) -> (-10.125, 56.5)
  line L41 (-10.125, 56.5) -> (-11, 56.5)
  line L42 (-11, 56.5) -> (-11, 55.5)
  line L43 (-11, 55.5) -> (-12, 55.5)
  line L44 (-12, 55.5) -> (-12, 56.5)
  line L45 (-12, 56.5) -> (-13, 56.5)
  line L46 (-13, 56.5) -> (-13, 53)
  line L47 (-13, 53) -> (15, 53)
  line L48 (15, 53) -> (15, 52)
  line L49 (15, 52) -> (100, 52)
  line L50 (100, 52) -> (100, -52)
  line L51 (100, -52) -> (15, -52)
  line L52 (15, -52) -> (15, -53)
  line L53 (15, -53) -> (-13, -53)
  line L54 (-13, -53) -> (-13, -56.5)
  line L55 (-13, -56.5) -> (-12, -56.5)
  line L56 (-12, -56.5) -> (-12, -55.5)
  line L57 (-12, -55.5) -> (-11, -55.5)
  line L58 (-11, -55.5) -> (-11, -56.5)
  line L59 (-11, -56.5) -> (-10.125, -56.5)
  line L60 (-10.125, -56.5) -> (-10.125, -55.5)
  line L61 (-10.125, -55.5) -> (-9.125, -55.5)
  line L62 (-9.125, -55.5) -> (-9.125, -56.5)
  line L63 (-9.125, -56.5) -> (-8.25, -56.5)
  line L64 (-13, 56.5) -> (-13, 58.5)
  line L65 (-3, 58.5) -> (0, 55)
  line L66 (-13, 58.5) -> (-11, 58.5)
  line L67 (-11, 58.5) -> (-11, 56.5)
  line L68 (-11, 56.5) -> (-9, 56.5)
  line L69 (-9, 56.5) -> (-9, 58.5)
  line L70 (-9, 58.5) -> (-7, 58.5)
  line L71 (-7, 58.5) -> (-7, 56.5)
  line L72 (-7, 56.5) -> (-5, 56.5)
  line L73 (-5, 56.5) -> (-5, 58.5)
  line L74 (-5, 58.5) -> (-3, 58.5)
  line L75 (0, 0) -> (26.4186, 0) construction
  line L76 (-13, -56.5) -> (-13, -58.5)
  line L77 (-13, -58.5) -> (-11, -58.5)
  line L78 (-11, -58.5) -> (-11, -56.5)
  line L79 (-11, -56.5) -> (-9, -56.5)
  line L80 (-9, -56.5) -> (-9, -58.5)
  line L81 (-9, -58.5) -> (-7, -58.5)
  line L82 (-7, -58.5) -> (-7, -56.5)
  line L83 (-7, -56.5) -> (-5, -56.5)
  line L84 (-5, -56.5) -> (-5, -58.5)
  line L85 (-5, -58.5) -> (-3, -58.5)
  line L86 (-3, -58.5) -> (0, -55)
  line L87 (-13, 56.5) -> (-15, 56.5)
  line L88 (-15, 56.5) -> (-15, 58.5)
  line L89 (-15, 58.5) -> (-17, 58.5)
  line L90 (-17, 58.5) -> (-17, 53)
  line L91 (-17, 53) -> (-13, 53)
  line L92 (-13, -56.5) -> (-15, -56.5)
  line L93 (-15, -56.5) -> (-15, -58.5)
  line L94 (-15, -58.5) -> (-17, -58.5)
  line L95 (-17, -58.5) -> (-17, -53)
  line L96 (-17, -53) -> (-13, -53)
  dimension "d401" = 2
  dimension "d402" = 2
  dimension "d403" = 2
  dimension "d404" = 2
  dimension "d405" = 2
  dimension "d406" = 2
  dimension "d407" = 2
  dimension "d408" = 2
  dimension "d409" = 2
  dimension "d410" = 2
  dimension "d411" = 2
  dimension "d412" = 2
  constraint coincident L45.end L46.start
  constraint perpendicular L45 L64
  constraint coincident L23.end L24.start
  constraint perpendicular L64 L66
  constraint perpendicular L66 L67
  constraint coincident L41.end L42.start
  constraint perpendicular L67 L68
  constraint perpendicular L68 L69
  constraint perpendicular L69 L70
  constraint perpendicular L70 L71
  constraint perpendicular L71 L72
  constraint perpendicular L72 L73
  constraint perpendicular L73 L74
  constraint coincident L75.start origin
  constraint perpendicular L46 L75
  constraint symmetric L45.end L75 L54.end
  constraint symmetric L64.end L75 L76.end
  constraint symmetric L65.start L75 L85.end
  constraint symmetric L23.end L75 L12.end
  constraint symmetric L66.end L75 L77.end
  constraint symmetric L41.end L75 L58.end
  constraint symmetric L68.end L75 L79.end
  constraint symmetric L69.end L75 L80.end
  constraint symmetric L70.end L75 L81.end
  constraint symmetric L71.end L75 L82.end
  constraint symmetric L72.end L75 L83.end
  constraint symmetric L73.end L75 L84.end
  constraint perpendicular L64 L87
  constraint perpendicular L87 L88
  constraint perpendicular L88 L89
  constraint perpendicular L47 L90
  constraint coincident L46.end L47.start
  constraint perpendicular L46 L91
  constraint symmetric L75 L87.end L92.end
  constraint symmetric L75 L88.end L93.end
  constraint symmetric L75 L89.end L94.end
  constraint symmetric L75 L90.end L95.end
  constraint symmetric L75 L46.end L53.end
  measures "d401" distance of L45.end L64.end
  measures "d402" distance of L64.end L66.end
  measures "d403" distance of L66.end L41.end
  measures "d404" distance of L41.end L68.end
  measures "d405" distance of L68.end L69.end
  measures "d406" distance of L69.end L70.end
  measures "d407" distance of L70.end L71.end
  measures "d408" distance of L71.end L72.end
  measures "d409" distance of L72.end L73.end
  measures "d410" distance of L45.end L87.end
  measures "d411" distance of L87.end L88.end
  measures "d412" distance of L88.end L89.end
extrude "Extrude18" add sketch "Grip Fix" against normal blind 5 contours L0 L1 L2 L3 L63 L80 L81 L82 | L60 L61 L62 L79 | L55 L56 L57 L58 L76 L77 L78 | L4 L5 L6 L83 | L7 L8 L9 L10 L11 L12 L84 L85 L86 | L54 L92 L93 L94 L95 L96 | L46 L87 L88 L89 L90 L91 | L42 L43 L44 L45 L64 L66 L67 | L38 L39 L40 L68 | L24 L25 L26 L27 L28 L29 L65 L73 L74 | L33 L34 L35 L36 L37 L69 L70 L71 | L30 L31 L32 L72 bodies 1 in component "Card Plate"